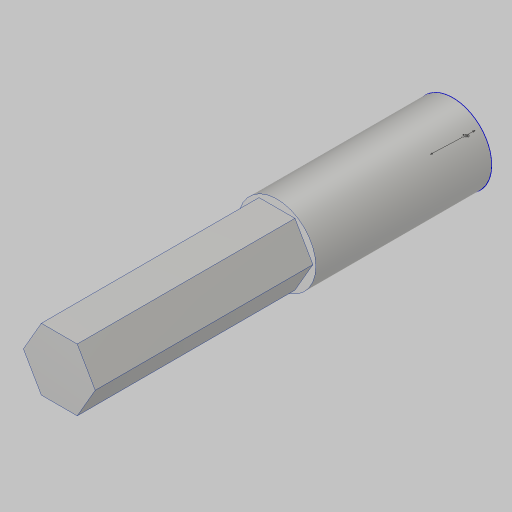
# Autodesk Inventor part: EL2-C2-002
Saved by Autodesk Inventor 2023.5 (Build 275446000, 446)
## iProperties
Created: 2025-02-14
Part Number: EL2-C2-002
Material: Aluminum 6061
Document SubType Name: Modeling
Designer: slick
Density: 2.7 g/cm^3
Appearance: Aluminum - Flat
Author: slick
Autodesk Inventor part; units mm, degrees
ref_plane "YZ Plane" through (0, 0, 0) normal (1, 0, 0) x (0, 1, 0)
ref_plane "XZ Plane" through (0, 0, 0) normal (0, 1, 0) x (-1, 0, 0)
ref_plane "XY Plane" through (0, 0, 0) normal (0, 0, 1) x (1, 0, 0)
sketch "Sketch1" plane through (0, 0, 0) normal (0, 0, 1) x (1, 0, 0)
  circle A0 centre (0, 0) radius 7.9375
  dimension "d0" = 15.875
  constraints: 1 centre point, 1 coincident
  measures "d0" diameter of A0
extrude "Extrusion1" add sketch "Sketch1" along normal mid plane 90.4875
sketch "Sketch2" plane through (0, 0, 45.2437) normal (0, 0, 1) x (1, 0, 0)
  line L0 (-3.6662, 6.35) -> (3.6662, 6.35)
  line L1 (3.6662, 6.35) -> (7.3323, 0)
  line L2 (7.3323, 0) -> (3.6662, -6.35)
  line L3 (3.6662, -6.35) -> (-3.6662, -6.35)
  line L4 (-3.6662, -6.35) -> (-7.3323, 0)
  line L5 (-7.3323, 0) -> (-3.6662, 6.35)
  circle A0 centre (0, 0) radius 7.9375 projected
  point P0 (0, -6.35)
  point P1 (0, 6.35)
  dimension "d3" = 12.7
  constraints: 12 end point, 2 midpoint, 1 coincident, 1 horizontal, 13 other
  measures "d3" distance of point (0, -6.35) point (0, 6.35)
extrude "Extrusion2" cut sketch "Sketch2" against normal blind 53.975
sketch "Sketch3" plane through (0, 0, 45.2437) normal (0, 0, 1) x (1, 0, 0)
  circle A0 centre (0, 0) radius 6.35
  circle A1 centre (0, 0) radius 7.9375 projected
  line L0 (3.6662, 6.35) -> (-3.6662, 6.35) projected
  line L1 (7.3323, 0) -> (3.6662, 6.35) projected
  line L2 (3.6662, -6.35) -> (7.3323, 0) projected
  line L3 (-3.6662, -6.35) -> (3.6662, -6.35) projected
  line L4 (-7.3323, 0) -> (-3.6662, -6.35) projected
  line L5 (-3.6662, 6.35) -> (-7.3323, 0) projected
  point P0 (-5.4993, 3.175)
  point P1 (0, 6.35)
  point P2 (-5.4993, -3.175)
  point P3 (0, -6.35)
  point P4 (5.4993, -3.175)
  point P5 (5.4993, 3.175)
  dimension "d6" = 12.7
  constraints: 1 centre point, 1 coincident
  measures "d6" diameter of A0
extrude "Extrusion3" cut sketch "Sketch3" against normal blind 6.35 contours A0 L1 L2 | A0 L0 L1 | L2 L3 A0 | A0 L5 L0 | L3 L4 A0 | A0 L4 L5
sketch "Sketch6" plane through (0, 0, 0) normal (1, 0, 0) x (0, 1, 0)
  line L0 (7.9375, -45.2437) -> (-7.9375, -45.2437) construction
  line L1 (-7.9375, -45.2437) -> (-7.9375, -8.7312) construction
  line L2 (-7.9375, -8.7312) -> (-6.35, -8.7312) construction
  line L3 (-6.35, -8.7312) -> (-6.35, 38.8938) construction
  line L4 (-6.35, 38.8938) -> (-6.35, 45.2437) construction
  line L5 (-6.35, 45.2437) -> (6.35, 45.2437) construction
  line L6 (6.35, 45.2437) -> (6.35, 38.8938) construction
  line L7 (6.35, 38.8938) -> (6.35, -8.7312) construction
  line L8 (6.35, -8.7312) -> (7.9375, -8.7312) construction
  line L9 (7.9375, -8.7312) -> (7.9375, -45.2437) construction
  line L10 (6.35, 45.2437) -> (-6.35, 45.2437)
  line L11 (-6.35, 45.2437) -> (-6.35, 35.7187)
  line L12 (-6.35, 35.7187) -> (6.35, 35.7188)
  line L13 (6.35, 35.7188) -> (6.35, 45.2437)
  line L14 (7.9375, -45.2437) -> (-7.9375, -45.2437)
  line L15 (-7.9375, -45.2437) -> (-7.9375, -44.6088)
  line L16 (-7.9375, -44.6088) -> (7.9375, -44.6088)
  line L17 (7.9375, -44.6088) -> (7.9375, -45.2437)
  point P0 (0, 0)
  dimension "d15" = 9.525
  dimension "d16" = 0.635
  constraints: 16 end point, 4 parallel, 4 point on line, 2 horizontal, 2 perpendicular
  measures "d15" distance of L12.end L10.start
  measures "d16" distance of L0.start L16.end
extrude "Extrusion6" cut sketch "Sketch6" along normal through all both and the other way through all
sketch "Sketch7" plane through (0, 0, -44.6088) normal (0, 0, -1) x (-1, 0, 0)
  circle A0 centre (0, 0) radius 6.35
  circle A1 centre (0, 0) radius 7.9375
  circle A2 centre (0, 0) radius 7.9375 construction
  dimension "d19" = 12.7
  constraints: 2 centre point, 2 coincident, 1 concentric
  measures "d19" diameter of A0
body "Solid1"
